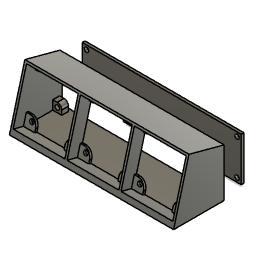
91c4-housing-3x (Autodesk Fusion 360 design; units mm, degrees)
Autodesk Fusion 360 part; units mm, degrees
sketch "스케치1" plane through (0, 0, 0) normal (0, 1, 0) x (1, 0, 0)
  line L0 (73, -26.5) -> (-73, -26.5)
  line L1 (-73, -26.5) -> (-73, 26.5)
  line L2 (-73, 26.5) -> (73, 26.5)
  line L3 (73, 26.5) -> (73, -26.5)
  line L4 (73, -26.5) -> (-73, 26.5) construction
  line L5 (-73, -26.5) -> (73, 26.5) construction
  line L6 (-25, -21.5) -> (-71, -21.5)
  line L7 (-71, -21.5) -> (-71, 24.5)
  line L8 (-71, 24.5) -> (-25, 24.5)
  line L9 (-25, 24.5) -> (-25, -21.5)
  line L10 (-25, -21.5) -> (-71, 24.5) construction
  line L11 (-71, -21.5) -> (-25, 24.5) construction
  line L12 (23, -21.5) -> (-23, -21.5)
  line L13 (-23, -21.5) -> (-23, 24.5)
  line L14 (-23, 24.5) -> (23, 24.5)
  line L15 (23, 24.5) -> (23, -21.5)
  line L16 (23, -21.5) -> (-23, 24.5) construction
  line L17 (-23, -21.5) -> (23, 24.5) construction
  line L18 (71, -21.5) -> (25, -21.5)
  line L19 (25, -21.5) -> (25, 24.5)
  line L20 (25, 24.5) -> (71, 24.5)
  line L21 (71, 24.5) -> (71, -21.5)
  line L22 (71, -21.5) -> (25, 24.5) construction
  line L23 (25, -21.5) -> (71, 24.5) construction
  point P0 (-48, 1.5)
  point P1 (0, 1.5)
  point P2 (48, 1.5)
  dimension "d1" = 146
  dimension "d2" = 53
  dimension "d3" = 46
  dimension "d4" = 46
  dimension "d5" = 2
  dimension "d6" = 2
  dimension "d7" = 46
  dimension "d8" = 46
  dimension "d9" = 2
  dimension "d10" = 46
  dimension "d11" = 46
  dimension "d12" = 2
  dimension "d13" = 5
  dimension "d130" = 2
  constraint horizontal L0
  constraint perpendicular L0 L1
  constraint parallel L0 L2
  constraint parallel L1 L3
  constraint coincident L4 origin
  constraint coincident L5 origin
  constraint horizontal L6
  constraint perpendicular L6 L7
  constraint parallel L6 L8
  constraint parallel L7 L9
  constraint coincident L10 P0
  constraint coincident L11 P0
  constraint horizontal L12
  constraint perpendicular L12 L13
  constraint parallel L12 L14
  constraint parallel L13 L15
  constraint coincident L16 P1
  constraint coincident L17 P1
  constraint collinear L8 L14
  constraint horizontal L18
  constraint perpendicular L18 L19
  constraint parallel L18 L20
  constraint parallel L19 L21
  constraint coincident L22 P2
  constraint coincident L23 P2
  constraint collinear L14 L20
  measures "d1" distance of L1.end L2.end
  measures "d2" distance of L0.end L1.end
  measures "d3" distance of L7.end L8.end
  measures "d4" distance of L6.end L7.end
  measures "d5" distance of L2 L8
  measures "d6" distance of L1 L7
  measures "d7" distance of L13.end L14.end
  measures "d8" distance of L12.end L13.end
  measures "d9" distance of L9 L13
  measures "d10" distance of L19.end L20.end
  measures "d11" distance of L18.end L19.end
  measures "d12" distance of L15 L19
  measures "d13" distance of L0 L6
  measures "d130" distance of L3 L21
extrude "돌출1" add sketch "스케치1" along normal blind 11.5 contours L0 L1 L2 L3 picked at (-7.666667, -24.833333) makes body 1
move_body "이동1" bodies 1 to x (1, 0, 0) y (0, 0.25881905, 0.96592583) z (0, -0.96592583, 0.25881905) at (0, 34.120615, 8.533148)
move_body "이동2" bodies 1 to x (1, 0, 0) y (0, 1, 0) z (0, 0, 1) at (0, -8.523581, 11.108147)
sketch "스케치2" plane through (0, 0, 0) normal (0, 1, 0) x (1, 0, 0)
  line L0 (-71, -24.408376) -> (-25, -24.408376)
  line L1 (-25, -24.408376) -> (-25, -36.314052)
  line L2 (-25, -36.314052) -> (-71, -36.314052)
  line L3 (-71, -36.314052) -> (-71, -24.408376)
  line L4 (-23, -24.408376) -> (23, -24.408376)
  line L5 (23, -24.408376) -> (23, -36.314052)
  line L6 (23, -36.314052) -> (-23, -36.314052)
  line L7 (-23, -36.314052) -> (-23, -24.408376)
  line L8 (25, -24.408376) -> (71, -24.408376)
  line L9 (71, -24.408376) -> (71, -36.314052)
  line L10 (71, -36.314052) -> (25, -36.314052)
  line L11 (25, -36.314052) -> (25, -24.408376)
  line L12 (73, -23.890738) -> (-73, -23.890738)
  line L13 (-73, -23.890738) -> (-73, -37.608147)
  line L14 (-73, -37.608147) -> (73, -37.608147)
  line L15 (73, -37.608147) -> (73, -23.890738)
extrude "돌출2" cut sketch "스케치2" along normal blind 2.976 contours L0 L1 L2 L3 | L4 L5 L6 L7 | L8 L9 L10 L11 | L12 L13 L14 L15 picked at (-40.333333, -28.376934) picked at (7.666667, -28.376934) picked at (55.666667, -32.345493) picked at (-72.333333, -32.604312) bodies 1
move_body "이동3" bodies 1 to x (1, 0, 0) y (0, 1, 0) z (0, 0, 1) at (0, -2.976, 0.797417)
sketch "스케치3" plane through (0, 6.625, 24.724837) normal (0, -0.258819, -0.965926) x (-1, 0, 0)
  line L0 (-73, -6.858705) -> (73, -6.858705)
  line L1 (73, -6.858705) -> (73, 43.060313)
  line L2 (73, 43.060313) -> (-73, 43.060313)
  line L3 (-73, 43.060313) -> (-73, -6.858705)
  line L4 (25, 41.060313) -> (71, 41.060313)
  line L5 (71, 41.060313) -> (71, -4.939687)
  line L6 (71, -4.939687) -> (25, -4.939687)
  line L7 (25, -4.939687) -> (25, 41.060313)
  line L8 (-23, 41.060313) -> (23, 41.060313)
  line L9 (23, 41.060313) -> (23, -4.939687)
  line L10 (23, -4.939687) -> (-23, -4.939687)
  line L11 (-23, -4.939687) -> (-23, 41.060313)
  line L12 (-71, 41.060313) -> (-25, 41.060313)
  line L13 (-25, 41.060313) -> (-25, -4.939687)
  line L14 (-25, -4.939687) -> (-71, -4.939687)
  line L15 (-71, -4.939687) -> (-71, 41.060313)
  circle A0 centre (-65, 1.060313) radius 2
  circle A1 centre (-31, 1.060313) radius 2
  circle A2 centre (-17, 1.060313) radius 2
  circle A3 centre (17, 1.060313) radius 2
  circle A4 centre (31, 1.060313) radius 2
  circle A5 centre (65, 1.060313) radius 2
  line L16 (-71, -4.939687) -> (-61, -4.939687)
  line L17 (-61, -4.939687) -> (-61, -1.939687)
  line L18 (-68, 5.060313) -> (-71, 5.060313)
  line L19 (-71, 5.060313) -> (-71, -4.939687)
  line L20 (-25, -4.939687) -> (-35, -4.939687)
  line L21 (-35, -4.939687) -> (-35, -1.939687)
  line L22 (-28, 5.060313) -> (-25, 5.060313)
  line L23 (-25, 5.060313) -> (-25, -4.939687)
  line L24 (-23, -4.939687) -> (-13, -4.939687)
  line L25 (-13, -4.939687) -> (-13, -1.939687)
  line L26 (-20, 5.060313) -> (-23, 5.060313)
  line L27 (-23, 5.060313) -> (-23, -4.939687)
  line L28 (23, -4.939687) -> (13, -4.939687)
  line L29 (13, -4.939687) -> (13, -1.939687)
  line L30 (20, 5.060313) -> (23, 5.060313)
  line L31 (23, 5.060313) -> (23, -4.939687)
  line L32 (25, -4.939687) -> (35, -4.939687)
  line L33 (35, -4.939687) -> (35, -1.939687)
  line L34 (28, 5.060313) -> (25, 5.060313)
  line L35 (25, 5.060313) -> (25, -4.939687)
  line L36 (71, -4.939687) -> (61, -4.939687)
  line L37 (61, -4.939687) -> (61, -1.939687)
  line L38 (68, 5.060313) -> (71, 5.060313)
  line L39 (71, 5.060313) -> (71, -4.939687)
  arc A6 (-61, -1.939687) -> (-68, 5.060313) centre (-68, -1.939687) ccw
  arc A7 (-28, 5.060313) -> (-35, -1.939687) centre (-28, -1.939687) ccw
  arc A8 (-13, -1.939687) -> (-20, 5.060313) centre (-20, -1.939687) ccw
  arc A9 (20, 5.060313) -> (13, -1.939687) centre (20, -1.939687) ccw
  arc A10 (35, -1.939687) -> (28, 5.060313) centre (28, -1.939687) ccw
  arc A11 (68, 5.060313) -> (61, -1.939687) centre (68, -1.939687) ccw
  line L40 (-71, 41.060313) -> (-65, 41.060313)
  line L41 (-65, 41.060313) -> (-65, 38.060313)
  line L42 (-68, 35.060313) -> (-71, 35.060313)
  line L43 (-71, 35.060313) -> (-71, 41.060313)
  line L44 (-25, 41.060313) -> (-31, 41.060313)
  line L45 (-31, 41.060313) -> (-31, 38.060313)
  line L46 (-28, 35.060313) -> (-25, 35.060313)
  line L47 (-25, 35.060313) -> (-25, 41.060313)
  line L48 (-23, 41.060313) -> (-17, 41.060313)
  line L49 (-17, 41.060313) -> (-17, 38.060313)
  line L50 (-20, 35.060313) -> (-23, 35.060313)
  line L51 (-23, 35.060313) -> (-23, 41.060313)
  line L52 (23, 41.060313) -> (17, 41.060313)
  line L53 (17, 41.060313) -> (17, 38.060313)
  line L54 (20, 35.060313) -> (23, 35.060313)
  line L55 (23, 35.060313) -> (23, 41.060313)
  line L56 (25, 41.060313) -> (31, 41.060313)
  line L57 (31, 41.060313) -> (31, 38.060313)
  line L58 (28, 35.060313) -> (25, 35.060313)
  line L59 (25, 35.060313) -> (25, 41.060313)
  line L60 (71, 41.060313) -> (65, 41.060313)
  line L61 (65, 41.060313) -> (65, 38.060313)
  line L62 (68, 35.060313) -> (71, 35.060313)
  line L63 (71, 35.060313) -> (71, 41.060313)
  arc A12 (65, 38.060313) -> (68, 35.060313) centre (68, 38.060313) ccw
  arc A13 (28, 35.060313) -> (31, 38.060313) centre (28, 38.060313) ccw
  arc A14 (17, 38.060313) -> (20, 35.060313) centre (20, 38.060313) ccw
  arc A15 (-20, 35.060313) -> (-17, 38.060313) centre (-20, 38.060313) ccw
  arc A16 (-31, 38.060313) -> (-28, 35.060313) centre (-28, 38.060313) ccw
  arc A17 (-68, 35.060313) -> (-65, 38.060313) centre (-68, 38.060313) ccw
  line L64 (-73, 43.060313) -> (-71, 43.060313)
  line L65 (-71, 43.060313) -> (-71, -4.939687)
  line L66 (-71, -4.939687) -> (-73, -4.939687)
  line L67 (-73, -4.939687) -> (-73, 43.060313)
  line L68 (73, 43.060313) -> (71, 43.060313)
  line L69 (71, 43.060313) -> (71, -4.939687)
  line L70 (71, -4.939687) -> (73, -4.939687)
  line L71 (73, -4.939687) -> (73, 43.060313)
  line L72 (-73, 43.060313) -> (73, 43.060313)
  line L73 (73, 43.060313) -> (73, 41.060313)
  line L74 (73, 41.060313) -> (-73, 41.060313)
  line L75 (-73, 41.060313) -> (-73, 43.060313)
  dimension "d19" = 4
  dimension "d21" = 6
  dimension "d22" = 4
  dimension "d24" = 6
  dimension "d26" = 34
  dimension "d27" = 4
  dimension "d29" = 6
  dimension "d30" = 4
  dimension "d32" = 6
  dimension "d33" = 4
  dimension "d35" = 6
  dimension "d36" = 4
  dimension "d38" = 6
  dimension "d39" = 10
  dimension "d40" = 10
  dimension "d41" = 10
  dimension "d42" = 10
  dimension "d43" = 10
  dimension "d44" = 10
  dimension "d45" = 10
  dimension "d46" = 10
  dimension "d47" = 10
  dimension "d48" = 10
  dimension "d49" = 10
  dimension "d50" = 10
  dimension "d51" = 7
  dimension "d52" = 6
  dimension "d53" = 6
  dimension "d54" = 6
  dimension "d55" = 6
  dimension "d56" = 6
  dimension "d57" = 6
  dimension "d58" = 6
  dimension "d59" = 6
  dimension "d60" = 6
  dimension "d61" = 6
  dimension "d62" = 6
  dimension "d63" = 6
  dimension "d64" = 3
  dimension "d71" = 2
  dimension "d131" = 6
  dimension "d132" = 6
  dimension "d133" = 6
  dimension "d134" = 6
  dimension "d135" = 6
  dimension "d136" = 6
  dimension "d137" = 146
  constraint horizontal L16
  constraint vertical L17
  constraint horizontal L18
  constraint vertical L19
  constraint horizontal L20
  constraint vertical L21
  constraint horizontal L22
  constraint vertical L23
  constraint horizontal L24
  constraint vertical L25
  constraint horizontal L26
  constraint vertical L27
  constraint horizontal L28
  constraint vertical L29
  constraint horizontal L30
  constraint vertical L31
  constraint horizontal L32
  constraint vertical L33
  constraint horizontal L34
  constraint vertical L35
  constraint horizontal L36
  constraint vertical L37
  constraint horizontal L38
  constraint vertical L39
  constraint tangent L17 A6
  constraint tangent L18 A6
  constraint tangent L21 A7
  constraint tangent L22 A7
  constraint equal A6 A7
  constraint tangent L25 A8
  constraint tangent L26 A8
  constraint equal A6 A8
  constraint tangent L29 A9
  constraint tangent L30 A9
  constraint equal A6 A9
  constraint tangent L33 A10
  constraint tangent L34 A10
  constraint equal A6 A10
  constraint tangent L37 A11
  constraint tangent L38 A11
  constraint equal A6 A11
  constraint horizontal L40
  constraint vertical L41
  constraint horizontal L42
  constraint vertical L43
  constraint horizontal L44
  constraint vertical L45
  constraint horizontal L46
  constraint vertical L47
  constraint horizontal L48
  constraint vertical L49
  constraint horizontal L50
  constraint vertical L51
  constraint horizontal L52
  constraint vertical L53
  constraint horizontal L54
  constraint vertical L55
  constraint horizontal L56
  constraint vertical L57
  constraint horizontal L58
  constraint vertical L59
  constraint horizontal L60
  constraint vertical L61
  constraint horizontal L62
  constraint vertical L63
  constraint tangent L61 A12
  constraint tangent L62 A12
  constraint tangent L57 A13
  constraint tangent L58 A13
  constraint equal A12 A13
  constraint tangent L53 A14
  constraint tangent L54 A14
  constraint equal A12 A14
  constraint tangent L49 A15
  constraint tangent L50 A15
  constraint equal A12 A15
  constraint tangent L45 A16
  constraint tangent L46 A16
  constraint equal A12 A16
  constraint tangent L41 A17
  constraint tangent L42 A17
  constraint equal A12 A17
  constraint horizontal L64
  constraint vertical L65
  constraint horizontal L66
  constraint vertical L67
  constraint horizontal L68
  constraint vertical L69
  constraint horizontal L70
  constraint vertical L71
  constraint horizontal L72
  constraint vertical L73
  constraint horizontal L74
  constraint vertical L75
  measures "d19" diameter of A0
  measures "d22" diameter of A1
  measures "d27" diameter of A2
  measures "d30" diameter of A3
  measures "d33" diameter of A4
  measures "d36" diameter of A5
  measures "d51" radius of A6
  measures "d64" radius of A12
  measures "d137" distance of L67 L73
extrude "돌출3" add sketch "스케치3" against normal blind 2 contours L14 L15 L16 L17 L18 L19 A6 L65 | L5 L6 L36 L37 L38 L39 A11 L69 | L12 L15 L40 L41 L42 L43 A17 L65 L74 | L4 L5 L60 L61 L62 L63 A12 L69 L74 | L13 L14 L20 L21 L22 L23 A7 | L6 L7 L32 L33 L34 L35 A10 | L12 L13 L44 L45 L46 L47 A16 L74 | L4 L7 L56 L57 L58 L59 A13 L74 | L8 L11 L48 L49 L50 L51 A15 L74 | L8 L9 L52 L53 L54 L55 A14 L74 | L10 L11 L24 L25 L26 L27 A8 | L9 L10 L28 L29 L30 L31 A9 picked at (-69.659221, 0.294285) picked at (69.659221, 0.294285) picked at (-68, 38.060313) picked at (68, 38.060313) picked at (-26.340779, 0.294285) picked at (26.340779, 0.294285) picked at (-28, 38.060313) picked at (28, 38.060313) picked at (-20, 38.060313) picked at (20, 38.060313) picked at (-21.659221, 0.294285) picked at (21.659221, 0.294285) bodies 1
sketch "스케치4" plane through (0, 0, 0) normal (0, 1, 0) x (1, 0, 0)
  line L0 (73, -26.5) -> (-73.4, -26.5)
  line L1 (-73.4, -26.5) -> (-73.4, 6.5)
  line L2 (-73.4, 6.5) -> (73, 6.5)
  line L3 (73, 6.5) -> (73, -26.5)
  point P0 (73, -26.5)
  dimension "d67" = 33
  constraint horizontal L0
  constraint vertical L1
  constraint horizontal L2
  constraint vertical L3
  constraint coincident P0 L0.start
  measures "d67" distance of P0 L2.end
extrude "돌출4" add sketch "스케치4" along normal blind 1.854 contours L0 L1 L2 L3 picked at (24.2, -15.5) bodies 1
sketch "스케치5" plane through (0, 1.854, 0) normal (0, 1, 0) x (-1, 0, 0)
  line L0 (-61, 26.003222) -> (-73, 26.003222)
  line L1 (-73, 26.003222) -> (-73, -6.5)
  line L2 (-73, -6.5) -> (73.4, -6.5)
  line L3 (73.4, -6.5) -> (73.4, 26.5)
  line L4 (73, 26.003222) -> (61, 26.003222)
  line L5 (61, 26.003222) -> (61, 26.004706)
  line L6 (61, 26.004706) -> (35, 26.004706)
  line L7 (35, 26.004706) -> (35, 26.003222)
  line L8 (35, 26.003222) -> (13, 26.003222)
  line L9 (13, 26.003222) -> (13, 26.004706)
  line L10 (13, 26.004706) -> (-13, 26.004706)
  line L11 (-13, 26.004706) -> (-13, 26.003222)
  line L12 (-13, 26.003222) -> (-35, 26.003222)
  line L13 (-35, 26.003222) -> (-35, 26.004706)
  line L14 (-35, 26.004706) -> (-61, 26.004706)
  line L15 (-61, 26.004706) -> (-61, 26.003222)
  line L16 (-73, -6.5) -> (73.4, -6.5)
  line L17 (73.4, -6.5) -> (73.4, -4.1)
  line L18 (73.4, -4.1) -> (-73, -4.1)
  line L19 (-73, -4.1) -> (-73, -6.5)
  line L20 (73.4, 26.5) -> (73, 26.5)
  line L21 (73, 26.5) -> (73, 26.003222)
  dimension "d70" = 2.4
  constraint horizontal L16
  constraint vertical L17
  constraint horizontal L18
  constraint vertical L19
  constraint coincident L1.end L2.start
  measures "d70" distance of L1.end L18.end
extrude "돌출5" add sketch "스케치3" along normal blind 32 contours L3 L15 L19 L43 L65 L66 L67 L74 | L1 L5 L39 L63 L69 L70 L71 L74 | L2 L3 L64 L65 L67 L72 L74 L75 | L1 L2 L68 L69 L71 L72 L73 L74 | L2 L4 L8 L12 L40 L44 L48 L52 L56 L60 L65 L69 L72 L74 picked at (-72.333333, 13.72698) picked at (72.333333, 23.72698) picked at (-72.333333, 42.393647) picked at (72.333333, 42.393647) picked at (5.666667, 42.393647) bodies 1
extrude "돌출6" add sketch "스케치5" along normal blind 40 contours L1 L2 L3 L16 L17 L18 L19 picked at (-24.2, -4.9) bodies 1
extrude "돌출7" cut sketch "스케치4" against normal blind 11 contours L0 L1 L2 L3 picked at (24.2, -15.5) bodies 1
sketch "스케치6" plane through (0, 0, -6.5) normal (0, 0, -1) x (-1, 0, 0)
  line L0 (-71, 40.767095) -> (-71, 0)
  line L1 (-71, 0) -> (71, 0)
  line L2 (71, 0) -> (71, 40.767095)
  line L3 (71, 40.767095) -> (-71, 40.767095)
  line L4 (78.000001, -5) -> (-83.000001, -5)
  line L5 (-83.000001, -5) -> (-83.000001, 58.000001)
  line L6 (-83.000001, 58.000001) -> (78.000001, 58.000001)
  line L7 (78.000001, 58.000001) -> (78.000001, -5)
  constraint horizontal L4
  constraint vertical L5
  constraint horizontal L6
  constraint vertical L7
extrude "돌출8" cut sketch "스케치6" along normal blind 41 contours L0 L1 L2 L3 | L4 L5 L6 L7 picked at (-23.666667, 27.178063) picked at (-25.333333, 52.255699) bodies 1
sketch "스케치8" plane through (0, 0, -4.1) normal (0, 0, 1) x (1, 0, 0)
  line L0 (-71, 41.410173) -> (-71, 1.854)
  line L1 (-71, 1.854) -> (71, 1.854)
  line L2 (71, 1.854) -> (71, 41.410173)
  line L3 (71, 41.410173) -> (-71, 41.410173)
  line L4 (-71, 1.854) -> (-63, 1.854)
  line L5 (-63, 1.854) -> (-63, 5.854)
  line L6 (-67, 9.854) -> (-71, 9.854)
  line L7 (-71, 9.854) -> (-71, 1.854)
  line L8 (-71, 41.410173) -> (-63, 41.410173)
  line L9 (-63, 41.410173) -> (-63, 37.410173)
  line L10 (-67, 33.410173) -> (-71, 33.410173)
  line L11 (-71, 33.410173) -> (-71, 41.410173)
  line L12 (71, 41.410173) -> (63, 41.410173)
  line L13 (63, 41.410173) -> (63, 37.410173)
  line L14 (67, 33.410173) -> (71, 33.410173)
  line L15 (71, 33.410173) -> (71, 41.410173)
  line L16 (71, 1.854) -> (63, 1.854)
  line L17 (63, 1.854) -> (63, 5.854)
  line L18 (67, 9.854) -> (71, 9.854)
  line L19 (71, 9.854) -> (71, 1.854)
  arc A0 (-67, 33.410173) -> (-63, 37.410173) centre (-67, 37.410173) ccw
  arc A1 (-63, 5.854) -> (-67, 9.854) centre (-67, 5.854) ccw
  arc A2 (67, 9.854) -> (63, 5.854) centre (67, 5.854) ccw
  arc A3 (63, 37.410173) -> (67, 33.410173) centre (67, 37.410173) ccw
  circle A4 centre (67, 5.854) radius 2
  line L20 (65.326397, 8.754411) -> (63.651369, 5.854823)
  line L21 (63.651369, 5.854823) -> (65.324972, 2.954411)
  line L22 (65.324972, 2.954411) -> (68.673603, 2.953589)
  line L23 (68.673603, 2.953589) -> (70.348631, 5.853177)
  line L24 (70.348631, 5.853177) -> (68.675028, 8.753589)
  line L25 (68.675028, 8.753589) -> (65.326397, 8.754411)
  circle A5 centre (67, 37.410173) radius 2
  line L26 (65.320464, 40.307152) -> (63.651374, 37.404142)
  line L27 (63.651374, 37.404142) -> (65.33091, 34.507162)
  line L28 (65.33091, 34.507162) -> (68.679536, 34.513193)
  line L29 (68.679536, 34.513193) -> (70.348626, 37.416204)
  line L30 (70.348626, 37.416204) -> (68.66909, 40.313184)
  line L31 (68.66909, 40.313184) -> (65.320464, 40.307152)
  circle A6 centre (-67, 37.410173) radius 2
  line L32 (-68.66909, 40.313184) -> (-70.348626, 37.416204)
  line L33 (-70.348626, 37.416204) -> (-68.679536, 34.513193)
  line L34 (-68.679536, 34.513193) -> (-65.33091, 34.507162)
  line L35 (-65.33091, 34.507162) -> (-63.651374, 37.404142)
  line L36 (-63.651374, 37.404142) -> (-65.320464, 40.307152)
  line L37 (-65.320464, 40.307152) -> (-68.66909, 40.313184)
  circle A7 centre (-67, 5.854) radius 2
  line L38 (-68.675028, 8.753589) -> (-70.348631, 5.853177)
  line L39 (-70.348631, 5.853177) -> (-68.673603, 2.953589)
  line L40 (-68.673603, 2.953589) -> (-65.324972, 2.954411)
  line L41 (-65.324972, 2.954411) -> (-63.651369, 5.854823)
  line L42 (-63.651369, 5.854823) -> (-65.326397, 8.754411)
  line L43 (-65.326397, 8.754411) -> (-68.675028, 8.753589)
  point P0 (67, 5.854)
  point P1 (67, 37.410173)
  point P2 (-67, 37.410173)
  point P3 (-67, 5.854)
  dimension "d82" = 8
  dimension "d83" = 8
  dimension "d84" = 8
  dimension "d85" = 8
  dimension "d86" = 8
  dimension "d87" = 8
  dimension "d88" = 8
  dimension "d89" = 8
  dimension "d90" = 4
  dimension "d95" = 4
  dimension "d96" = 2.9
  dimension "d97" = 4
  dimension "d98" = 2.9
  dimension "d99" = 4
  dimension "d100" = 2.9
  dimension "d101" = 4
  dimension "d102" = 2.9
  constraint horizontal L4
  constraint vertical L5
  constraint horizontal L6
  constraint vertical L7
  constraint coincident L0.end L1.start
  constraint horizontal L8
  constraint vertical L9
  constraint horizontal L10
  constraint vertical L11
  constraint horizontal L12
  constraint vertical L13
  constraint horizontal L14
  constraint vertical L15
  constraint horizontal L16
  constraint vertical L17
  constraint horizontal L18
  constraint vertical L19
  constraint coincident L1.end L2.start
  constraint tangent L9 A0
  constraint tangent L10 A0
  constraint tangent L5 A1
  constraint tangent L6 A1
  constraint equal A0 A1
  constraint tangent L17 A2
  constraint tangent L18 A2
  constraint equal A0 A2
  constraint tangent L13 A3
  constraint tangent L14 A3
  constraint equal A0 A3
  constraint concentric A2 A4
  constraint coincident P0 A2.centre
  constraint concentric A3 A5
  constraint concentric A0 A6
  constraint concentric A1 A7
  constraint coincident P3 A1.centre
  measures "d82" distance of L0.end L4.end
  measures "d83" distance of L0.end L6.end
  measures "d88" distance of L1.end L16.end
  measures "d89" distance of L1.end L18.end
  measures "d90" radius of A0
  measures "d95" diameter of A4
  measures "d96" distance of P0 L25
  measures "d97" diameter of A5
  measures "d99" diameter of A6
  measures "d101" diameter of A7
  measures "d102" distance of P3 L43
extrude "돌출10" add sketch "스케치8" along normal blind 6 contours L0 L3 L8 L9 L10 L11 A0 | L0 L1 L4 L5 L6 L7 A1 | L2 L3 L12 L13 L14 L15 A3 | L1 L2 L16 L17 L18 L19 A2 | A4 | L20 L21 L22 L23 L24 L25 | A5 | L26 L27 L28 L29 L30 L31 | A6 | L32 L33 L34 L35 L36 L37 | A7 | L38 L39 L40 L41 L42 L43 picked at (-70.005905, 39.713187) picked at (-70.007412, 3.553589) picked at (70.005905, 39.713187) picked at (70.007412, 3.553589) picked at (66.214604, 5.400552) picked at (69.275199, 7.109511) picked at (66.119391, 36.927355) picked at (64.7233, 38.663078) picked at (-67.880609, 36.927355) picked at (-69.223398, 38.7554) picked at (-67.785396, 5.400552) picked at (-69.224904, 4.511375) bodies 1
extrude "돌출11" cut sketch "스케치8" against normal blind 20 contours L0 L3 L8 L9 L10 L11 A0 | L0 L1 L2 L3 L5 L6 L9 L10 L13 L14 L17 L18 A0 A1 A2 A3 | L0 L1 L4 L5 L6 L7 A1 | L2 L3 L12 L13 L14 L15 A3 | L1 L2 L16 L17 L18 L19 A2 | A4 | L20 L21 L22 L23 L24 L25 | A5 | L26 L27 L28 L29 L30 L31 | A6 | L32 L33 L34 L35 L36 L37 | A7 | L38 L39 L40 L41 L42 L43 picked at (-70.005905, 39.713187) picked at (21.054009, 26.515805) picked at (-70.007412, 3.553589) picked at (70.005905, 39.713187) picked at (70.007412, 3.553589) picked at (66.214604, 5.400552) picked at (69.275199, 7.109511) picked at (66.119391, 36.927355) picked at (64.7233, 38.663078) picked at (-67.880609, 36.927355) picked at (-69.223398, 38.7554) picked at (-67.785396, 5.400552) picked at (-69.224904, 4.511375) bodies 1
extrude "돌출12" cut sketch "스케치8" along normal blind 7 contours A4 | A5 | A6 | A7 picked at (66.214604, 5.400552) picked at (66.119391, 36.927355) picked at (-67.880609, 36.927355) picked at (-67.785396, 5.400552) bodies 1
extrude "돌출13" cut sketch "스케치8" along normal blind 3 contours L20 L21 L22 L23 L24 L25 | L26 L27 L28 L29 L30 L31 | L32 L33 L34 L35 L36 L37 | L38 L39 L40 L41 L42 L43 picked at (69.275199, 7.109511) picked at (64.7233, 38.663078) picked at (-69.223398, 38.7554) picked at (-69.224904, 4.511375) bodies 1
extrude "돌출14" add 2 faces at (-65.666667, 41.410173, -0.1) (68.333333, 41.410173, -2.1) along direction (0, 1, 0) blind 2 on bodies 1 bodies 1
extrude "돌출15" add sketch "스케치8" against normal blind 2.4 separate body contours L0 L3 L8 L9 L10 L11 A0 | L0 L1 L2 L3 L5 L6 L9 L10 L13 L14 L17 L18 A0 A1 A2 A3 | L0 L1 L4 L5 L6 L7 A1 | L2 L3 L12 L13 L14 L15 A3 | L1 L2 L16 L17 L18 L19 A2 | L20 L21 L22 L23 L24 L25 | L26 L27 L28 L29 L30 L31 | L32 L33 L34 L35 L36 L37 | L38 L39 L40 L41 L42 L43 picked at (-70.005905, 39.713187) picked at (21.054009, 26.515805) picked at (-70.007412, 3.553589) picked at (70.005905, 39.713187) picked at (70.007412, 3.553589) picked at (69.275199, 7.109511) picked at (64.7233, 38.663078) picked at (-69.223398, 38.7554) picked at (-69.224904, 4.511375) makes body 2
move_body "이동4" bodies 2 to x (1, 0, 0) y (0, 1, 0) z (0, 0, 1) at (0, 0, -20)
sketch "스케치9" plane through (0, 0, -24.1) normal (0, 0, 1) x (1, 0, 0)
  circle A0 centre (67, 37.410173) radius 2
  circle A1 centre (67, 5.854) radius 2
  circle A2 centre (-67, 37.410173) radius 2
  circle A3 centre (-67, 5.854) radius 2
  line L0 (71, 1.854) -> (71, 41.410173)
  line L1 (71, 41.410173) -> (-71, 41.410173)
  line L2 (-71, 41.410173) -> (-71, 1.854)
  line L3 (-71, 1.854) -> (71, 1.854)
  line L4 (-27.4, 6.954) -> (-21, 6.954)
  line L5 (-21, 3.354) -> (-27.4, 3.354)
  line L6 (-18.2, 2.424) -> (-30.2, 2.424)
  line L7 (-30.2, 2.424) -> (-30.2, 8.084)
  line L8 (-30.2, 8.084) -> (-18.2, 8.084)
  line L9 (-18.2, 8.084) -> (-18.2, 2.424)
  line L10 (-27.4, 6.954) -> (-21, 3.354) construction
  line L11 (-27.4, 3.354) -> (-21, 6.954) construction
  arc A4 (-27.4, 6.954) -> (-27.4, 3.354) centre (-27.4, 5.154) ccw
  arc A5 (-21, 3.354) -> (-21, 6.954) centre (-21, 5.154) ccw
  point P0 (-24.2, 5.154)
  point P1 (-24.2, 5.154)
  dimension "d115" = 46.8
  dimension "d124" = 1.5
  dimension "d125" = 12
  dimension "d145" = 6.4
  dimension "d146" = 3.6
  constraint horizontal L5
  constraint horizontal L4
  constraint horizontal L6
  constraint perpendicular L6 L7
  constraint parallel L6 L8
  constraint parallel L7 L9
  constraint midpoint L10 P1
  constraint coincident P1 P0
  constraint vertical L4.start L5.end
  constraint vertical L5.start L4.end
  constraint tangent L4 A4
  constraint tangent L4 A5
  measures "d115" distance of L2 P1
  measures "d124" distance of L3 L5
  measures "d125" distance of L7.end L8.end
  measures "d145" distance of L4.end L4.start
  measures "d146" distance of L4 L5
extrude "돌출16" cut 3 faces at (-71, 38.743506, -24.9) (-71, 25.558115, -24.9) (-71, 7.187333, -24.9) along direction (1, 0, 0) blind 0.3 on bodies 2 bodies 2
extrude "돌출17" cut 1 faces at (-23.466667, 41.410173, -24.9) along direction (0, -1, 0) blind 0.3 on bodies 2 bodies 2
extrude "돌출18" cut 1 faces at (23.766667, 1.854, -24.9) along direction (0, 1, 0) blind 0.3 on bodies 2 bodies 2
extrude "돌출19" cut 1 faces at (71, 15.139391, -24.9) along direction (-1, 0, 0) blind 0.3 on bodies 2 bodies 2
extrude "돌출20" cut sketch "스케치9" against normal blind 3 contours L4 L5 A4 A5 picked at (-25.266667, 4.554) bodies 2
extrude "돌출21" add sketch "스케치9" along normal blind 4 contours L4 L5 A4 A5 | L6 L7 L8 L9 picked at (-25.266667, 4.554) picked at (-25.266667, 7.707333) bodies 2
extrude "돌출9" cut sketch "스케치8" against normal blind 23 contours L0 L3 L8 L9 L10 L11 A0 | L0 L1 L2 L3 L5 L6 L9 L10 L13 L14 L17 L18 A0 A1 A2 A3 | L0 L1 L4 L5 L6 L7 A1 | L2 L3 L12 L13 L14 L15 A3 | L1 L2 L16 L17 L18 L19 A2 | A4 | L20 L21 L22 L23 L24 L25 | A5 | L26 L27 L28 L29 L30 L31 | A6 | L32 L33 L34 L35 L36 L37 | A7 | L38 L39 L40 L41 L42 L43 picked at (-70.005905, 39.713187) picked at (21.054009, 26.515805) picked at (-70.007412, 3.553589) picked at (70.005905, 39.713187) picked at (70.007412, 3.553589) picked at (66.214604, 5.400552) picked at (69.275199, 7.109511) picked at (66.119391, 36.927355) picked at (64.7233, 38.663078) picked at (-67.880609, 36.927355) picked at (-69.223398, 38.7554) picked at (-67.785396, 5.400552) picked at (-69.224904, 4.511375) bodies 1
extrude "돌출22" cut 1 faces at (-73.4, 14.569333, -5.7) along direction (1, 0, 0) blind 0.2 on bodies 1 bodies 1
extrude "돌출23" cut 1 faces at (-73.2, 14.569333, -5.7) along direction (1, 0, 0) blind 0.2 on bodies 1 bodies 1
extrude "돌출24" cut sketch "스케치9" along normal blind 7 contours L4 L5 A4 A5 picked at (-25.266667, 4.554) bodies 2
